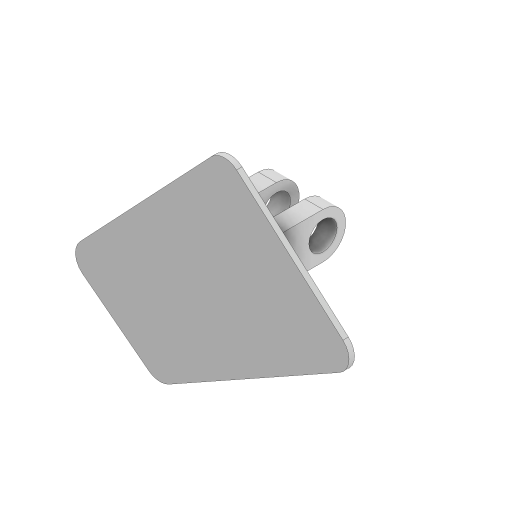
# Autodesk Inventor part: Upper Back Plate
Saved by Autodesk Inventor 2024 (Build 280153000, 153)
## iProperties
Created: 2025-04-26
Part Number: Upper Back Plate
Material: Generic
Document SubType Name: Modeling
Designer: Binara
Density: 1 g/cm^3
Appearance: Default
Author: Binara
Autodesk Inventor part; units mm, degrees
ref_plane "YZ Plane" through (0, 0, 0) normal (1, 0, 0) x (0, 1, 0)
ref_plane "XZ Plane" through (0, 0, 0) normal (0, 1, 0) x (-1, 0, 0)
ref_plane "XY Plane" through (0, 0, 0) normal (0, 0, 1) x (1, 0, 0)
sketch "Sketch1" plane through (0, 0, 0) normal (0, 0, 1) x (1, 0, 0)
  line L0 (22.1506, 55.679) -> (98.2363, -11.7464)
  line L1 (98.2363, -11.7464) -> (-13.4178, -74.2233)
  line L2 (-13.4178, -74.2233) -> (-63.8323, -35.4735)
  line L3 (-63.8323, -35.4735) -> (22.1506, 55.679)
  point P0 (0, 0)
  constraints: 8 end point
extrude "Extrusion1" add sketch "Sketch1" along normal blind 3
fillet "Fillet1" radius 10 4 edges at (98.2363, -11.7464, 1.5) (-13.4178, -74.2233, 1.5) (22.1506, 55.679, 1.5) (-63.8323, -35.4735, 1.5)
sketch "Sketch2" plane through (0, 0, 0) normal (0, 0, -1) x (-1, 0, 0)
  line L0 (-41.2625, -6.2798) -> (-5.7625, -6.2798)
  line L1 (-5.7625, -6.2798) -> (-5.7625, 18.7202)
  line L2 (-5.7625, 18.7202) -> (-41.2625, 18.7202)
  line L3 (-41.2625, 18.7202) -> (-41.2625, -6.2798)
  line L4 (-41.2625, -6.2798) -> (-5.7625, 18.7202) construction
  line L5 (-5.7625, -6.2798) -> (-41.2625, 18.7202) construction
  line L6 (-31.2625, -6.2798) -> (-15.7625, -6.2798)
  line L7 (-15.7625, -6.2798) -> (-15.7625, 18.7202)
  line L8 (-15.7625, 18.7202) -> (-31.2625, 18.7202)
  line L9 (-31.2625, 18.7202) -> (-31.2625, -6.2798)
  line L10 (-31.2625, -6.2798) -> (-15.7625, 18.7202) construction
  line L11 (-15.7625, -6.2798) -> (-31.2625, 18.7202) construction
  point P0 (0, 0)
  point P1 (-23.5125, 6.2202)
  point P2 (-31.2625, -6.2798)
  point P3 (-15.7625, -6.2798)
  dimension "d3" = 10
  dimension "d4" = 25
  dimension "d8" = 15.5
  constraints: 24 end point, 4 midpoint, 4 parallel, 2 horizontal, 2 perpendicular, 1 point on line
  measures "d3" distance between parallel lines of L1 L7
  measures "d4" distance of L2.end L0.start
  measures "d8" distance between parallel lines of L9 L7
extrude "Extrusion2" add sketch "Sketch2" along normal blind 45 contours L3 L2 L9 L0 | L7 L2 L1 L0
fillet "Fillet2" radius 12.5 4 edges at (10.7625, 18.7202, -45) (36.2625, 18.7202, -45) (10.7625, -6.2798, -45) (36.2625, -6.2798, -45)
sketch "Sketch3" plane through (5.7625, -6.2798, 0) normal (-1, 0, 0) x (0, 0, 1)
  arc A0 (-32.5, 25) -> (-32.5, 0) centre (-32.5, 12.5) ccw projected
  circle A1 centre (-32.5, 12.5) radius 7.75
  point P0 (0, 6.2798)
  dimension "d9" = 15.5
  constraints: 1 centre point, 1 coincident
  measures "d9" diameter of A1
extrude "Extrusion3" cut sketch "Sketch3" against normal up to surface (35.5 mm away)
fillet "Fillet3" radius 5 4 edges at (5.7625, 6.2202, 0) (10.7625, 18.7202, 0) (41.2625, 6.2202, 0) (36.2625, 18.7202, 0)
body "Solid1"
